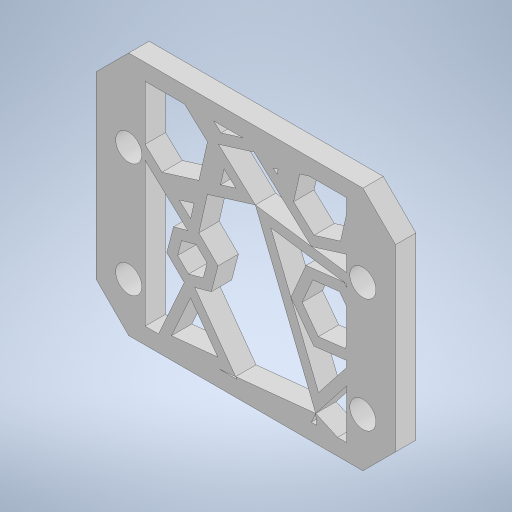
# Autodesk Inventor part: министена
Saved by Autodesk Inventor 2023.1 (Build 271208000, 208)
## iProperties
Created: 2025-12-15
Part Number: министена
Material: Типовые
Document SubType Name: Modeling
Designer: DELL
Density: 1 g/cm^3
Appearance: По умолчанию
Author: DELL
Autodesk Inventor part; units mm, degrees
ref_plane "YZ Plane" through (0, 0, 0) normal (1, 0, 0) x (0, 1, 0)
ref_plane "XZ Plane" through (0, 0, 0) normal (0, 1, 0) x (-1, 0, 0)
ref_plane "XY Plane" through (0, 0, 0) normal (0, 0, 1) x (1, 0, 0)
sketch "Эскиз1" plane through (0, 0, 0) normal (0, 0, 1) x (1, 0, 0)
  line L0 (-4.2707, -4.9523) -> (-2.3077, -4.7523)
  line L1 (-2.3077, -4.7523) -> (-2.1633, -4.9523)
  line L2 (-11.3118, -6.8759) -> (-11.3461, -6.9523)
  line L3 (-11.7634, -4.9523) -> (-8.0812, 3.2477)
  line L4 (-8.0812, 3.2477) -> (-2.3077, -4.7523)
  line L5 (-2.3077, -4.7523) -> (-4.2707, -4.9523)
  line L6 (-10.1765, -4.3478) -> (-4.4971, -3.7692)
  line L7 (-4.4971, -3.7692) -> (-7.8379, 0.86)
  line L8 (-7.8379, 0.86) -> (-10.1765, -4.3478)
  line L9 (-2.3077, -4.7523) -> (7.5073, -3.7523)
  line L10 (7.5073, -3.7523) -> (6.9684, -4.9523)
  line L11 (-6.7622, 21.0477) -> (-4.4071, 18.8658)
  line L12 (-4.4071, 18.8658) -> (-5.7718, 12.8658)
  line L13 (-7.1851, 12.4287) -> (-10.4105, 11.4311)
  line L14 (-5.7718, 12.8658) -> (-7.1365, 6.8658)
  line L15 (-7.1365, 6.8658) -> (-11.6503, 11.0477)
  line L16 (-10.4105, 11.4311) -> (-7.1851, 12.4287)
  line L17 (-7.4029, 11.1053) -> (-7.8262, 9.2439)
  line L18 (-7.8262, 9.2439) -> (-9.2236, 10.5421)
  line L19 (-5.7718, 12.8658) -> (-4.4071, 18.8658)
  line L20 (-4.4071, 18.8658) -> (0.1067, 14.684)
  line L21 (0.1067, 14.684) -> (-5.7718, 12.8658)
  line L22 (-2.2854, 15.2681) -> (-4.1564, 14.6894)
  line L23 (-3.7221, 16.5991) -> (-2.2854, 15.2681)
  line L24 (-3.7221, 16.5991) -> (-4.1564, 14.6894)
  line L25 (-7.4029, 11.1053) -> (-9.2236, 10.5421)
  line L26 (-5.7718, 12.8658) -> (-7.1851, 12.4287)
  line L27 (-10.4105, 11.4311) -> (-11.4141, 11.1207)
  line L28 (7.5073, -3.7523) -> (0.1067, 14.684)
  line L29 (11.2859, 1.0617) -> (7.5073, -3.7523)
  line L30 (1.9946, 13.2022) -> (11.2859, 11.875)
  line L31 (7.8466, -1.3764) -> (1.9946, 13.2022)
  line L32 (0.1067, 14.684) -> (11.2859, 13.0872)
  line L33 (11.2859, 3.7623) -> (7.2772, 3.2858)
  line L34 (7.2772, 3.2858) -> (4.465, 7.0478)
  line L35 (4.465, 7.0478) -> (6.3169, 11.3642)
  line L36 (6.3169, 11.3642) -> (10.981, 11.9186)
  line L37 (10.981, 11.9186) -> (11.2859, 11.5107)
  line L38 (7.8235, 4.5592) -> (11.1116, 4.9501)
  line L39 (11.1116, 4.9501) -> (11.2859, 5.3562)
  line L40 (11.2859, 9.5064) -> (10.4346, 10.6452)
  line L41 (10.4346, 10.6452) -> (7.1465, 10.2543)
  line L42 (7.1465, 10.2543) -> (5.841, 7.2113)
  line L43 (5.841, 7.2113) -> (7.8235, 4.5592)
  line L44 (7.5073, -3.7523) -> (7.6295, -4.9523)
  line L45 (7.5073, -3.7523) -> (10.1796, -4.9523)
  line L46 (-4.0997, 20.2169) -> (-1.4136, 21.0477)
  line L47 (-4.0997, 20.2169) -> (-4.9965, 21.0477)
  line L48 (6.9877, 13.7011) -> (3.472, 16.9583)
  line L49 (3.472, 16.9583) -> (4.4021, 21.0477)
  line L50 (11.2723, 21.0477) -> (11.2859, 21.0351)
  line L51 (11.2859, 15.0305) -> (6.9877, 13.7011)
  line L52 (11.3055, 19.3811) -> (9.5066, 21.0477)
  line L53 (6.7083, 21.0477) -> (5.5514, 20.6898)
  line L54 (5.5514, 20.6898) -> (4.7958, 17.3677)
  line L55 (4.7958, 17.3677) -> (7.295, 15.0523)
  line L56 (7.295, 15.0523) -> (10.5499, 16.059)
  line L57 (10.5499, 16.059) -> (11.3055, 19.3811)
  line L58 (11.2859, 13.8843) -> (11.1103, 13.1123)
  line L59 (4.4021, 21.0477) -> (3.472, 16.9583)
  line L60 (3.472, 16.9583) -> (-0.0437, 20.2154)
  line L61 (-0.0437, 20.2154) -> (2.6472, 21.0477)
  line L62 (6.9877, 13.7011) -> (11.1103, 13.1123)
  line L63 (-0.0437, 20.2154) -> (0.1067, 14.684)
  line L64 (1.1878, 19.0745) -> (1.3118, 14.5119)
  line L65 (2.2965, 19.6831) -> (2.9039, 19.871)
  line L66 (2.7629, 19.2511) -> (2.2965, 19.6831)
  line L67 (2.7629, 19.2511) -> (2.9039, 19.871)
  line L68 (-8.0812, 3.2477) -> (-9.4117, 4.5613)
  line L69 (-9.4117, 4.5613) -> (-8.9393, 6.3704)
  line L70 (-8.9393, 6.3704) -> (-7.1365, 6.8658)
  line L71 (-7.1365, 6.8658) -> (-5.8059, 5.5522)
  line L72 (-5.8059, 5.5522) -> (-6.2783, 3.7431)
  line L73 (-6.2783, 3.7431) -> (-8.0812, 3.2477)
  line L74 (-6.8232, 8.2429) -> (-4.4698, 5.9194)
  line L75 (-4.4698, 5.9194) -> (-5.2923, 2.7696)
  line L76 (-5.2923, 2.7696) -> (-7.3317, 2.2091)
  line L77 (-8.1724, 7.8256) -> (-9.9254, 7.3439)
  line L78 (-9.9254, 7.3439) -> (-10.7478, 4.1941)
  line L79 (-10.7478, 4.1941) -> (-8.6058, 2.0793)
  line L80 (-19.4141, -6.9523) -> (-19.4141, 23.0477)
  line L81 (-19.4141, -6.9523) -> (-19.4141, 23.0477)
  line L82 (-4.4071, 18.8658) -> (2.6472, 21.0477)
  line L83 (17.2859, 23.0477) -> (17.2859, -6.9523)
  line L84 (-19.4141, -6.9523) -> (17.2859, -6.9523)
  line L85 (-19.4141, 23.0477) -> (17.2859, 23.0477)
  line L86 (10.2859, 20.2698) -> (-12.4141, -4.1745) construction
  line L87 (-12.4141, 20.2698) -> (10.2859, -4.1745) construction
  line L88 (11.2859, 3.0053) -> (7.8466, -1.3764)
  line L89 (11.2859, 21.0477) -> (-13.4141, 21.0477)
  line L90 (-13.4141, 21.0477) -> (-13.4141, -4.9523)
  line L91 (-13.4141, -4.9523) -> (11.2859, -4.9523)
  line L92 (11.2859, -4.9523) -> (11.2859, 21.0477)
  line L93 (11.2859, 21.0477) -> (-13.4141, -4.9523) construction
  line L94 (-13.4141, 21.0477) -> (11.2859, -4.9523) construction
  line L95 (-6.8095, 13.8272) -> (-11.3365, 12.427)
  line L96 (-11.3365, 12.427) -> (-13.4141, 14.3518)
  line L97 (-13.4141, 20.3756) -> (-11.2413, 21.0477)
  line L98 (-8.5648, 21.0477) -> (-5.7586, 18.4478)
  line L99 (-5.7586, 18.4478) -> (-6.8095, 13.8272)
  line L100 (-5.7718, 12.8658) -> (-11.6503, 11.0477)
  line L101 (-11.6503, 11.0477) -> (-13.4141, 12.6818)
  line L102 (-6.7622, 21.0477) -> (-4.4071, 18.8658)
  line L103 (-4.4071, 18.8658) -> (-5.7718, 12.8658)
  point P0 (0, 0)
  point P1 (-7.5038, -2.419)
  point P2 (-10.2856, 17.0477)
  point P3 (-8.1862, 10.2598)
  point P4 (-3.3574, 15.4719)
  point P5 (9.1291, 7.6022)
  point P6 (9.1291, 7.6022)
  point P7 (8.0506, 18.3744)
  point P8 (2.6544, 19.6017)
  point P9 (4.465, 7.0478)
  point P10 (4.465, 7.0478)
  point P11 (10.981, 11.9186)
  point P12 (10.981, 11.9186)
  point P13 (11.5663, 15.1173)
  point P14 (-7.6088, 5.0568)
  point P15 (-1.0641, 8.0477)
  point P16 (-10.2856, 17.0477)
  point P17 (-10.2856, 17.0477)
  point P18 (11.2859, 19.3992)
  dimension "d39" = 1.2
  dimension "d40" = 1.2
  dimension "d47" = 6
  dimension "d49" = 1.2
  dimension "d53" = 1.2
  dimension "d74" = 1.2
  dimension "d84" = 1.2
  dimension "d85" = 1.2
  dimension "d86" = 60
  dimension "d87" = 60
  dimension "d90" = 1.2
  dimension "d100" = 1.2
  dimension "d109" = 1.2
  dimension "d117" = 1.2
  dimension "d118" = 1.2
  dimension "d156" = 30
  dimension "d159" = 24.7
  dimension "d166" = 6
  constraints: 208 end point, 17 point on line, 13 parallel, 4 midpoint, 3 coincident, 3 perpendicular, 2 collinear, 1 horizontal, 1 vertical, 73 other
  measures "d39" distance between parallel lines of L4 L7
  measures "d40" distance between parallel lines of L3 L8
  measures "d47" vertical distance of L11.end L12.end
  measures "d49" distance between parallel lines of L14 L17
  measures "d53" distance between parallel lines of L13 L25
  measures "d74" distance between parallel lines of L33 L38
  measures "d84" distance between parallel lines of L28 L31
  measures "d85" distance between parallel lines of L30 L32
  measures "d86" angle of L29 L32
  measures "d87" angle of L28 L32
  measures "d90" distance between parallel lines of L11 L47
  measures "d100" distance between parallel lines of L50 L52
  measures "d109" distance between parallel lines of L63 L64
  measures "d117" distance between parallel lines of L71 L74
  measures "d118" distance between parallel lines of L70 L77
  measures "d156" distance of L83.start L83.end
  measures "d159" distance of L91.end L90.end
  measures "d166" distance between parallel lines of L81 L90
extrude "Выдавливание1" add sketch "Эскиз1" along normal blind 2.5 contours L91 L3 L4 L0 | L9 L10 L91 L1 | L4 L73 L72 L71 L14 L74 L75 L76 | L28 L32 L92 L30 L31 L88 L29 | L45 L91 L44 | L79 L78 L77 L15 L70 L69 L68 L3 | L21 L12 L20 | L90 L96 L95 L99 L98 L89 L11 L12 L26 L13 L27 L100 L101 | L11 L89 L47 L46 L61 L82 | L14 L15 L100 L27 L13 L26 | L61 L89 L49 L60 | L48 L49 L89 L53 L54 L55 L56 L57 L92 L51 | L33 L34 L35 L36 L37 L92 L40 L41 L42 L43 L38 L39 | L80 L85 L83 L84
sketch "Эскиз2" plane through (0, 0, 2.5) normal (0, 0, 1) x (1, 0, 0)
  line L0 (-19.4141, 23.0477) -> (-19.4141, -6.9523) construction
  line L1 (-15.4141, 25.0477) -> (-15.4141, -8.9523) construction
  circle A0 centre (-15.4141, 13.0477) radius 1.6
  circle A1 centre (-15.4141, -0.9523) radius 1.6
  circle A2 centre (13.2859, 13.0477) radius 1.6
  circle A3 centre (13.2859, -0.9523) radius 1.6
  line L2 (17.2859, -6.9523) -> (17.2859, 23.0477) projected
  line L3 (17.2859, 23.0477) -> (-19.4141, 23.0477) projected
  point P0 (0, 0)
  point P1 (18.0359, 25.0477)
  point P2 (18.0359, -8.9523)
  dimension "d128" = 3.2
  dimension "d129" = 3.2
  dimension "d132" = 14
  dimension "d139" = 4
  dimension "d140" = 4
  dimension "d151" = 14
  dimension "d152" = 4
  dimension "d153" = 10
  dimension "d154" = 10
  constraints: 4 centre point, 2 end point, 2 point on line, 1 vertical
  measures "d128" diameter of A0
  measures "d129" diameter of A1
  measures "d132" distance of A1.centre A0.centre
  measures "d139" distance from line of L2 A2.centre
  measures "d140" distance from line of L2 A3.centre
  measures "d151" distance of A2.centre A3.centre
  measures "d152" distance between parallel lines of L0 L1
  measures "d153" distance from line of L3 A0.centre
  measures "d154" distance from line of L3 A2.centre
extrude "Выдавливание2" cut sketch "Эскиз2" against normal blind 2.5
chamfer "Фаска1" distance 4 angle 45 4 edges at (-19.4141, 23.0477, 1.25) (17.2859, 23.0477, 1.25) (17.2859, -6.9523, 1.25) (-19.4141, -6.9523, 1.25)
